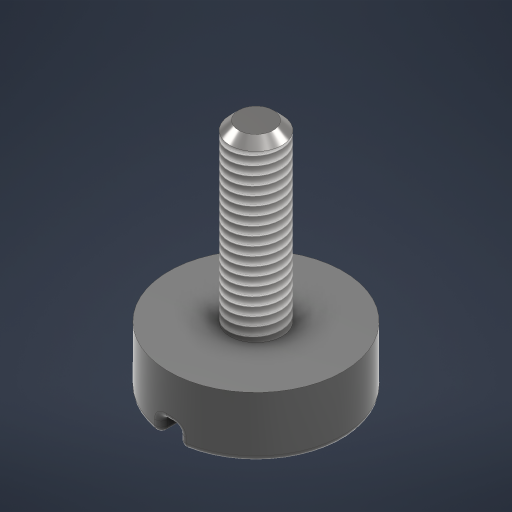
# Autodesk Inventor part: M6x1 Feet
Saved by Autodesk Inventor 2023 (Build 270158000, 158)
## iProperties
Created: 2023-03-05
Part Number: M6x1 Feet
Material: Stainless Steel
Document SubType Name: Modeling
Designer: roota
Density: 8 g/cm^3
Appearance: Semi-Polished
Author: roota
Autodesk Inventor part; units mm, degrees
ref_plane "YZ Plane" through (0, 0, 0) normal (1, 0, 0) x (0, 1, 0)
ref_plane "XZ Plane" through (0, 0, 0) normal (0, 1, 0) x (-1, 0, 0)
ref_plane "XY Plane" through (0, 0, 0) normal (0, 0, 1) x (1, 0, 0)
sketch "Sketch1" plane through (0, 0, 0) normal (0, 1, 0) x (-1, 0, 0)
  circle A0 centre (0, 0) radius 3
  dimension "d0" = 6
  constraints: 1 centre point, 1 coincident
  measures "d0" diameter of A0
extrude "Extrusion1" add sketch "Sketch1" along normal blind 20
sketch "Sketch2" plane through (0, 0, 0) normal (0, -1, 0) x (1, 0, 0)
  circle A0 centre (0, 0) radius 10
  dimension "d3" = 20
  constraints: 1 centre point, 1 coincident
  measures "d3" diameter of A0
extrude "Extrusion2" add sketch "Sketch2" along normal blind 7
chamfer "Chamfer1" distance 1 angle 45 1 edges at (3, 20, 0)
sketch "Sketch3" plane through (0, -7, 0) normal (0, -1, 0) x (1, 0, 0)
  line L0 (-1, 12.4438) -> (1, 12.4438)
  line L1 (1, 12.4438) -> (1, -12.4438)
  line L2 (1, -12.4438) -> (-1, -12.4438)
  line L3 (-1, -12.4438) -> (-1, 12.4438)
  line L4 (-1, 12.4438) -> (1, -12.4438) construction
  line L5 (1, 12.4438) -> (-1, -12.4438) construction
  point P0 (0, 0)
  dimension "d9" = 2
  constraints: 12 end point, 2 midpoint, 2 parallel, 1 horizontal, 1 perpendicular
  measures "d9" distance of L1.end L2.end
extrude "Extrusion3" cut sketch "Sketch3" against normal blind 2
fillet "Fillet1" radius 0.7 13 edges at (-10, -7, 0) (7.4162, -7, -6.7082) (7.4162, -7, 6.7082) (1, -7, 0) (1, -6, -9.9499) (1, -6, 9.9499) (1, -5, 0) (0, -5, -10) (0, -5, 10) (-1, -5, 0) (-1, -6, -9.9499) (-1, -6, 9.9499) (-1, -7, 0)
thread "Thread1" size "M6x1" class "6g" standard "ISO Metric profile" length 20
body "Solid1"
